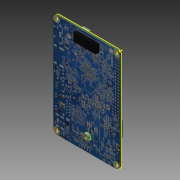
# Autodesk Inventor part: nanopc_t4
Saved by Autodesk Inventor 2013 SP2 (Build 170200200, 200)
## iProperties
Created: 2018-09-03
Part Number: nanopc_t4
Material: Generic
Document SubType Name: Modeling
Designer: alex
Density: 1 g/cm^3
Author: alex
Autodesk Inventor part; units mm, degrees
ref_plane "YZ Plane" through (0, 0, 0) normal (1, 0, 0) x (0, 1, 0)
ref_plane "XZ Plane" through (0, 0, 0) normal (0, 1, 0) x (-1, 0, 0)
ref_plane "XY Plane" through (0, 0, 0) normal (0, 0, 1) x (1, 0, 0)
sketch "Sketch1" plane through (0, 0, 0) normal (0, 1, 0) x (-1, 0, 0)
  line L0 (0, 0) -> (64, 0)
  line L1 (64, 0) -> (64, -100)
  line L2 (64, -100) -> (0, -100)
  line L3 (0, -100) -> (0, 0)
  dimension "d0" = 64
  dimension "d1" = 100
  constraints: 8 end point, 2 parallel, 1 horizontal, 1 perpendicular
  measures "d0" distance of L1.end L2.end
  measures "d1" distance of L0.end L1.end
extrude "Extrusion1" add sketch "Sketch1" along normal blind 1.8
fillet "Fillet1" radius 4 4 edges at (-64, 0.9, 0) (0, 0.9, 0) (0, 0.9, -100) (-64, 0.9, -100)
sketch "Sketch2" plane through (0, 0, 0) normal (0, -1, 0) x (1, 0, 0)
  arc A0 (-64, -96) -> (-60, -100) centre (-60, -96) ccw projected
  arc A1 (-4, -100) -> (0, -96) centre (-4, -96) ccw projected
  arc A2 (0, -4) -> (-4, 0) centre (-4, -4) ccw projected
  arc A3 (-60, 0) -> (-64, -4) centre (-60, -4) ccw projected
  line L0 (-64, -4) -> (-64, -96) projected
  line L1 (-60, -100) -> (-60, -96)
  line L2 (-60, -96) -> (-64, -96)
  line L3 (0, -96) -> (-4, -96)
  line L4 (-4, -96) -> (-4, -100)
  line L5 (0, -4) -> (-4, -4)
  line L6 (-4, -4) -> (-4, 0)
  line L7 (-60, 0) -> (-60, -4)
  line L8 (-60, -4) -> (-64, -4)
  point P0 (0, 0)
  point P1 (-60.8, -96.8)
  point P2 (-3.2, -96.8)
  point P3 (-3.2, -3.2)
  point P4 (-60.8, -3.2)
  dimension "d5" = 4
  dimension "d6" = 0.8
  dimension "d7" = 0.8
  dimension "d8" = 0.8
  dimension "d9" = 0.8
  dimension "d10" = 0.8
  dimension "d11" = 0.8
  dimension "d12" = 0.8
  dimension "d13" = 0.8
  constraints: 16 end point, 5 perpendicular, 2 parallel
  measures "d5" distance of L1.start L1.end
  measures "d6" distance from line of L2 point (-60.8, -96.8)
  measures "d7" distance from line of L1 point (-60.8, -96.8)
  measures "d8" distance from line of L3 point (-3.2, -96.8)
  measures "d9" distance from line of L4 point (-3.2, -96.8)
  measures "d10" distance from line of L5 point (-3.2, -3.2)
  measures "d11" distance from line of L6 point (-3.2, -3.2)
  measures "d12" distance from line of L8 point (-60.8, -3.2)
  measures "d13" distance from line of L7 point (-60.8, -3.2)
hole "Hole1" at (-60.8, 0, -96.8) at (-3.2, 0, -96.8) at (-3.2, 0, -3.2) at (-60.8, 0, -3.2) direction (0, 1, 0) diameter 3.2 end through all
sketch "Sketch3" plane through (0, 1.8, 0) normal (0, 1, 0) x (1, 0, 0)
  line L0 (-24.0749, 86.9532) -> (-9.798, 86.9532)
  line L1 (-9.798, 86.9532) -> (-9.798, 74.9855)
  line L2 (-9.798, 74.9855) -> (-24.0749, 74.9855)
  line L3 (-24.0749, 74.9855) -> (-24.0749, 86.9532)
  line L4 (-42.004, 76.8088) -> (-36.0181, 76.8088)
  line L5 (-36.0181, 76.8088) -> (-36.0181, 71.0747)
  line L6 (-36.0181, 71.0747) -> (-42.004, 71.0747)
  line L7 (-42.004, 71.0747) -> (-42.004, 76.8088)
  line L8 (-26.0395, 59.4207) -> (-18.9932, 59.4207)
  line L9 (-18.9932, 59.4207) -> (-18.9932, 52.191)
  line L10 (-18.9932, 52.191) -> (-26.0395, 52.191)
  line L11 (-26.0395, 52.191) -> (-26.0395, 59.4207)
  line L12 (-21.1941, 72.0637) -> (-16.9365, 72.0637)
  line L13 (-16.9365, 72.0637) -> (-16.9365, 67.1402)
  line L14 (-16.9365, 67.1402) -> (-21.1941, 67.1402)
  line L15 (-21.1941, 67.1402) -> (-21.1941, 72.0637)
  line L16 (-31.5453, 82.6589) -> (-26.0395, 82.6589)
  line L17 (-26.0395, 82.6589) -> (-26.0395, 77.9216)
  line L18 (-26.0395, 77.9216) -> (-31.5453, 77.9216)
  line L19 (-31.5453, 77.9216) -> (-31.5453, 82.6589)
  line L20 (-27.0702, 92.6857) -> (-6.8232, 92.6857)
  line L21 (-6.8232, 92.6857) -> (-6.8232, 89.4983)
  line L22 (-6.8232, 89.4983) -> (-27.0702, 89.4983)
  line L23 (-27.0702, 89.4983) -> (-27.0702, 92.6857)
  line L24 (-27.0702, 97.7771) -> (-6.9471, 97.7771)
  line L25 (-6.9471, 97.7771) -> (-6.9471, 94.5771)
  line L26 (-6.9471, 94.5771) -> (-27.0702, 94.5771)
  line L27 (-27.0702, 94.5771) -> (-27.0702, 97.7771)
  line L28 (-27.0702, 9.0883) -> (-6.8232, 9.0883)
  line L29 (-6.8232, 9.0883) -> (-6.8232, 11.9431)
  line L30 (-6.8232, 11.9431) -> (-27.0702, 11.9431)
  line L31 (-27.0702, 11.9431) -> (-27.0702, 9.0883)
  line L32 (-28.1635, 5.4758) -> (-8.1648, 5.4758)
  line L33 (-8.1648, 5.4758) -> (-8.1648, 2.1639)
  line L34 (-8.1648, 2.1639) -> (-28.1635, 2.1639)
  line L35 (-28.1635, 2.1639) -> (-28.1635, 5.4758)
  line L36 (-39.5623, 5.4758) -> (-32.7683, 5.4758)
  line L37 (-32.7683, 5.4758) -> (-32.7683, 1.1716)
  line L38 (-32.7683, 1.1716) -> (-39.5623, 1.1716)
  line L39 (-39.5623, 1.1716) -> (-39.5623, 5.4758)
  line L40 (-55.1326, 3.3237) -> (-50.3337, 3.3237)
  line L41 (-50.3337, 3.3237) -> (-50.3337, 0.6285)
  line L42 (-50.3337, 0.6285) -> (-55.1326, 0.6285)
  line L43 (-55.1326, 0.6285) -> (-55.1326, 3.3237)
  line L44 (-47.0326, 0.6285) -> (-42.004, 0.6285)
  line L45 (-42.004, 0.6285) -> (-42.004, 3.3237)
  line L46 (-42.004, 3.3237) -> (-47.0326, 3.3237)
  line L47 (-47.0326, 3.3237) -> (-47.0326, 0.6285)
  line L48 (-55.1326, 96.8) -> (-50.3337, 96.8)
  line L49 (-50.3337, 96.8) -> (-50.3337, 99.4879)
  line L50 (-50.3337, 99.4879) -> (-55.1326, 99.4879)
  line L51 (-55.1326, 99.4879) -> (-55.1326, 96.8)
  point P0 (0, 0)
  constraints: 104 end point, 26 parallel, 13 horizontal, 13 perpendicular, 1 point on line
extrude "Extrusion2" add sketch "Sketch3" along normal blind 1 contours L0 L1 L2 L3 | L4 L5 L6 L7 | L8 L9 L10 L11 | L12 L13 L14 L15 | L16 L17 L18 L19 | L32 L33 L34 L35
extrude "Extrusion3" add sketch "Sketch3" along normal blind 3 contours L20 L21 L22 L23 | L24 L25 L26 L27 | L31 L30 L29 L28
extrude "Extrusion4" add sketch "Sketch3" along normal blind 1 contours L40 L41 L42 L43 | L47 L46 L45 L44 | L51 L50 L49 L48
extrude "Extrusion5" add sketch "Sketch3" along normal blind 3 contours L36 L37 L38 L39
sketch "Sketch4" plane through (0, 1.8, 0) normal (0, 1, 0) x (1, 0, 0)
  line L0 (-32.7683, 5.4758) -> (-32.7683, 1.1716) projected
  line L1 (-32.7683, 1.1716) -> (-39.5623, 1.1716) projected
  line L2 (-39.5623, 1.1716) -> (-39.5623, 5.4758) projected
  line L3 (-39.5623, 5.4758) -> (-32.7683, 5.4758) projected
  line L4 (-50.3337, 3.3237) -> (-50.3337, 0.6285) projected
  line L5 (-50.3337, 0.6285) -> (-55.1326, 0.6285) projected
  line L6 (-55.1326, 0.6285) -> (-55.1326, 3.3237) projected
  line L7 (-55.1326, 3.3237) -> (-50.3337, 3.3237) projected
  line L8 (-55.1326, 96.8) -> (-55.1326, 99.4879) projected
  line L9 (-55.1326, 99.4879) -> (-50.3337, 99.4879) projected
  line L10 (-50.3337, 99.4879) -> (-50.3337, 96.8) projected
  line L11 (-50.3337, 96.8) -> (-55.1326, 96.8) projected
  line L12 (-47.0326, 0.6285) -> (-47.0326, 3.3237) projected
  line L13 (-47.0326, 3.3237) -> (-42.004, 3.3237) projected
  line L14 (-42.004, 3.3237) -> (-42.004, 0.6285) projected
  line L15 (-42.004, 0.6285) -> (-47.0326, 0.6285) projected
  line L16 (-6.9471, 97.7771) -> (-6.9471, 94.5771) projected
  line L17 (-6.9471, 94.5771) -> (-27.0702, 94.5771) projected
  line L18 (-27.0702, 94.5771) -> (-27.0702, 97.7771) projected
  line L19 (-27.0702, 97.7771) -> (-6.9471, 97.7771) projected
  line L20 (-27.0702, 9.0883) -> (-27.0702, 11.9431) projected
  line L21 (-27.0702, 11.9431) -> (-6.8232, 11.9431) projected
  line L22 (-6.8232, 11.9431) -> (-6.8232, 9.0883) projected
  line L23 (-6.8232, 9.0883) -> (-27.0702, 9.0883) projected
  line L24 (-6.8232, 92.6857) -> (-6.8232, 89.4983) projected
  line L25 (-6.8232, 89.4983) -> (-27.0702, 89.4983) projected
  line L26 (-27.0702, 89.4983) -> (-27.0702, 92.6857) projected
  line L27 (-27.0702, 92.6857) -> (-6.8232, 92.6857) projected
  line L28 (-8.1648, 5.4758) -> (-8.1648, 2.1639) projected
  line L29 (-8.1648, 2.1639) -> (-28.1635, 2.1639) projected
  line L30 (-28.1635, 2.1639) -> (-28.1635, 5.4758) projected
  line L31 (-28.1635, 5.4758) -> (-8.1648, 5.4758) projected
  line L32 (-36.0181, 76.8088) -> (-36.0181, 71.0747) projected
  line L33 (-36.0181, 71.0747) -> (-42.004, 71.0747) projected
  line L34 (-42.004, 71.0747) -> (-42.004, 76.8088) projected
  line L35 (-42.004, 76.8088) -> (-36.0181, 76.8088) projected
  line L36 (-16.9365, 72.0637) -> (-16.9365, 67.1402) projected
  line L37 (-16.9365, 67.1402) -> (-21.1941, 67.1402) projected
  line L38 (-21.1941, 67.1402) -> (-21.1941, 72.0637) projected
  line L39 (-21.1941, 72.0637) -> (-16.9365, 72.0637) projected
  line L40 (-26.0395, 82.6589) -> (-26.0395, 77.9216) projected
  line L41 (-26.0395, 77.9216) -> (-31.5453, 77.9216) projected
  line L42 (-31.5453, 77.9216) -> (-31.5453, 82.6589) projected
  line L43 (-31.5453, 82.6589) -> (-26.0395, 82.6589) projected
  line L44 (-18.9932, 59.4207) -> (-18.9932, 52.191) projected
  line L45 (-18.9932, 52.191) -> (-26.0395, 52.191) projected
  line L46 (-26.0395, 52.191) -> (-26.0395, 59.4207) projected
  line L47 (-26.0395, 59.4207) -> (-18.9932, 59.4207) projected
  line L48 (-9.798, 86.9532) -> (-9.798, 74.9855) projected
  line L49 (-9.798, 74.9855) -> (-24.0749, 74.9855) projected
  line L50 (-24.0749, 74.9855) -> (-24.0749, 86.9532) projected
  line L51 (-24.0749, 86.9532) -> (-9.798, 86.9532) projected
  circle A0 centre (-3.2, 3.2) radius 1.6 projected
  circle A1 centre (-60.8, 96.8) radius 1.6 projected
  circle A2 centre (-3.2, 96.8) radius 1.6 projected
  circle A3 centre (-60.8, 3.2) radius 1.6 projected
  arc A4 (-60, 100) -> (-64, 96) centre (-60, 96) ccw projected
  line L52 (-64, 96) -> (-64, 4) projected
  arc A5 (-64, 4) -> (-60, 0) centre (-60, 4) ccw projected
  line L53 (-60, 0) -> (-4, 0) projected
  arc A6 (-4, 0) -> (0, 4) centre (-4, 4) ccw projected
  line L54 (0, 4) -> (0, 96) projected
  arc A7 (0, 96) -> (-4, 100) centre (-4, 96) ccw projected
  line L55 (-4, 100) -> (-60, 100) projected
  point P0 (0, 0)
sketch "Sketch5" plane through (0, 1.8, 0) normal (0, 1, 0) x (1, 0, 0)
  line L0 (-51.5216, 14.0163) -> (-8.0501, 14.0163)
  line L1 (-8.0501, 14.0163) -> (-8.0501, 50.2303)
  line L2 (-8.0501, 50.2303) -> (-51.5216, 50.2303)
  line L3 (-51.5216, 50.2303) -> (-51.5216, 14.0163)
  line L4 (-51.5216, 50.2303) -> (-45.958, 50.2303)
  line L5 (-45.958, 50.2303) -> (-45.958, 45.2733)
  line L6 (-45.958, 45.2733) -> (-51.5216, 45.2733)
  line L7 (-51.5216, 45.2733) -> (-51.5216, 50.2303)
  circle A0 centre (-48.6054, 11.1502) radius 2.866
  line L8 (-51.5216, 14.0163) -> (-51.471, 11.1006)
  arc A1 (-43.4561, 14.0163) -> (-45.7398, 11.1006) centre (-43.2203, 11.4794) ccw
  circle A2 centre (-10.5958, 52.7257) radius 2.4954
  line L9 (-8.0501, 50.2303) -> (-8.1009, 52.7756)
  arc A3 (-16.0357, 50.2303) -> (-13.0911, 52.7088) centre (-16.6158, 53.908) ccw
  point P0 (0, 0)
  constraints: 20 end point, 8 point on circle, 4 centre point, 4 parallel, 4 tangent, 2 horizontal, 2 perpendicular, 2 point on line
extrude "Extrusion6" add sketch "Sketch5" along normal blind 8 contours L0 L3 L6 L5 L2 L1 | A1 A0 L0 | A0 L8 L0 | A0 A1 | L2 A2 L9 | L2 A3 A2 | A2 picked at (-49.5355, 10.9245)
sketch "Sketch7" plane through (0, 0, 0) normal (0, -1, 0) x (1, 0, 0)
  line L0 (-41.7523, -3.2) -> (-19.972, -3.2)
  line L1 (-19.972, -3.2) -> (-19.972, -11.1201)
  line L2 (-19.972, -11.1201) -> (-41.7523, -11.1201)
  line L3 (-41.7523, -11.1201) -> (-41.7523, -3.2)
  point P0 (0, 0)
  constraints: 8 end point, 2 parallel, 1 horizontal, 1 perpendicular
extrude "Extrusion7" add sketch "Sketch7" along normal blind 3
sketch "Sketch8" plane through (0, 0, 0) normal (0, -1, 0) x (1, 0, 0)
  circle A0 centre (-30.8621, -86.2682) radius 2.9892
  point P0 (0, 0)
  constraints: 1 centre point
extrude "Extrusion8" add sketch "Sketch8" along normal blind 2
sketch "Sketch9" plane through (-30.8621, -2, -86.2682) normal (0, -1, 0) x (1, 0, 0)
  circle A0 centre (0, 0) radius 2.9892 projected
  point P0 (30.8621, 86.2682)
hole "Hole2" at (-30.8621, -2, -86.2682) direction (0, 1, 0) diameter 3.2 end through all
sketch "Sketch10" plane through (0, 1.8, 0) normal (0, 1, 0) x (1, 0, 0)
  line L0 (0, 4) -> (0, 96) projected
  line L1 (0, 73.518) -> (-14.2183, 73.518)
  line L2 (-14.2183, 73.518) -> (-14.2183, 58.9192)
  line L3 (-14.2183, 58.9192) -> (0, 58.9192)
  line L4 (0, 58.9192) -> (0, 73.518)
  point P0 (0, 0)
  constraints: 8 end point, 2 parallel, 1 horizontal, 1 perpendicular, 1 point on line
extrude "Extrusion9" add sketch "Sketch10" along normal blind 1
body "Solid1"
